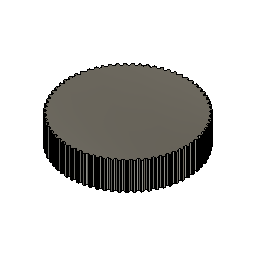
gear_69z (Autodesk Fusion 360 design; units mm, degrees)
Autodesk Fusion 360 part; units mm, degrees
sketch "Sketch1" plane through (0, 0, 0) normal (0, 0, 1) x (1, 0, 0) in component "gt2 pulley"
  circle A0 centre (0, 0) radius 21.9634 construction
  circle A1 centre (0, 0) radius 20.9594 construction
  line L0 (0, 0) -> (0, 21.9634) construction
  line L1 (0, 0) -> (0.9997, 21.9406) construction
  line L2 (0, 0) -> (1.4056, 21.9184) construction
  circle A2 centre (0, 0) radius 21.7094 construction
  arc A3 (0.3936, 21.5719) -> (0.4678, 21.2766) centre (1.3893, 21.6649) ccw
  circle A4 centre (0, 0) radius 21.5594 construction
  arc A5 (0.2459, 21.708) -> (0, 21.7094) centre (0, 0) ccw
  arc A6 (0.3936, 21.5719) -> (0.2459, 21.708) centre (0.2443, 21.558) ccw
  arc A7 (0.4678, 21.2766) -> (0.954, 20.9377) centre (0.9792, 21.4921) ccw
  arc A8 (0, 21.7094) -> (-0.2459, 21.708) centre (0, 0) ccw
  arc A9 (-0.2459, 21.708) -> (-0.3936, 21.5719) centre (-0.2443, 21.558) ccw
  arc A10 (-0.4678, 21.2766) -> (-0.3936, 21.5719) centre (-1.3893, 21.6649) ccw
  arc A11 (-0.954, 20.9377) -> (-0.4678, 21.2766) centre (-0.9792, 21.4921) ccw
  arc A12 (0.954, 20.9377) -> (-0.954, 20.9377) centre (0, 0) ccw
  point P0 (1.3893, 21.6649)
  point P1 (0, 21.7094)
  dimension "d18" = 43.9268
  dimension "d19" = 2.609
  dimension "d22" = 1.004
  dimension "d24" = 0.75
  dimension "d26" = 1
  dimension "d27" = 0.15
  dimension "d28" = 0.15
  dimension "d47" = 0.555
  dimension "d52" = 3.812
  constraint coincident A0.centre A1.centre
  constraint coincident A0 L0.end
  constraint vertical L0
  constraint coincident A0 L1.end
  constraint coincident A0 L2.end
  constraint concentric A1 A2
  constraint coincident A1 A7.end
  constraint coincident L1 A7.end
  constraint coincident A2 P0
  constraint coincident L2 P0
  constraint coincident P0 A3.centre
  constraint coincident A2 P1
  constraint coincident L0 P1
  constraint concentric A2 A4
  constraint coincident P1 A5.end
  constraint coincident A4 A6.centre
  constraint coincident A3.start A6.start
  constraint tangent A3 A6
  constraint tangent A3 A7
  constraint symmetric L0 A7.end A11.start
  constraint symmetric L0 A3.start A9.end
  constraint symmetric L0 A3.end A10.start
  constraint symmetric L0 A3 A10
  constraint symmetric L0 A5.start A8.end
  constraint symmetric L0 P1 A5.end
  constraint symmetric L0 A5 A8
  constraint symmetric L0 A6 A9
  constraint symmetric L0 A7 A11
  constraint coincident A1 A11.start
  constraint tangent A1 A7
  constraint coincident L1 A7.centre
  measures "d18" diameter of A0
  measures "d19" angle of L0 L1
  measures "d22" distance of A0 A1
  measures "d24" distance of A1 A2
  measures "d26" radius of A3
  measures "d27" distance of A2 A4
  measures "d28" radius of A6
  measures "d47" radius of A7
extrude "Extrude1" add sketch "Sketch1" along normal blind 10 makes body 1
pattern_circular "C-Pattern1" count 69 over 360 about axis through (0, 0, 1.75) along (0, 0, 1) of bodies 1 makes body 2 at (-1.1657, 20.9269, 3.3333) makes body 3 at (-3.9003, 20.5933, 6.6667) makes body 4 at (-6.3658, 19.9693, 6.6667) makes body 5 at (-8.1553, 19.3077, 6.6667) makes body 6 at (-9.8773, 18.4861, 6.6667) makes body 7 at (-10.9806, 17.8528, 6.6667) makes body 8 at (-13.062, 16.3914, 6.6667) makes body 9 at (-13.391, 16.1238, 3.3333) makes body 10 at (-15.6748, 13.9139, 6.6667) makes body 11 at (-17, 12.2595, 6.6667) makes body 12 at (-18.0444, 10.6628, 6.6667) makes body 13 at (-18.9393, 8.9778, 6.6667) makes body 14 at (-19.117, 8.5927, 3.3333) makes body 15 at (-20.2521, 5.3991, 6.6667) makes body 16 at (-20.3572, 4.9882, 3.3333) makes body 17 at (-20.7264, 3.1163, 3.3333) makes body 18 at (-20.9239, 1.2187, 6.6667) makes body 19 at (-20.903, -1.5361, 6.6667) makes body 20 at (-20.7104, -3.2212, 6.6667) makes body 21 at (-20.3317, -5.0911, 6.6667) makes body 22 at (-19.9853, -6.3152, 3.3333) makes body 23 at (-19.0733, -8.6893, 6.6667) makes body 24 at (-17.7689, -11.1158, 6.6667) makes body 25 at (-17.5404, -11.473, 3.3333) makes body 26 at (-16.4244, -13.0205, 6.6667) makes body 27 at (-15.1723, -14.4601, 3.3333) makes body 28 at (-13.7946, -15.7799, 3.3333) makes body 29 at (-12.3025, -16.969, 3.3333) makes body 30 at (-9.9707, -18.4359, 6.6667) makes body 31 at (-7.8614, -19.4292, 6.6667) makes body 32 at (-5.8587, -20.1239, 6.6667) makes body 33 at (-5.4503, -20.2383, 3.3333) makes body 34 at (-3.5873, -20.6501, 3.3333) makes body 35 at (-1.6947, -20.8908, 3.3333) makes body 36 at (1.6947, -20.8908, 6.6667) makes body 37 at (3.5873, -20.6501, 6.6667) makes body 38 at (4.8336, -20.3944, 6.6667) makes body 39 at (7.2681, -19.6589, 6.6667) makes body 40 at (8.8338, -19.0068, 6.6667) makes body 41 at (10.1567, -18.3341, 6.6667) makes body 42 at (11.7818, -17.3345, 6.6667) makes body 43 at (13.3093, -16.1913, 6.6667) makes body 44 at (14.111, -15.4976, 3.3333) makes body 45 at (15.4618, -14.1502, 6.6667) makes body 46 at (17.1841, -12.0001, 6.6667) makes body 47 at (17.7689, -11.1158, 3.3333) makes body 48 at (18.7061, -9.4539, 6.6667) makes body 49 at (19.9853, -6.3152, 6.6667) makes body 50 at (20.2791, -5.2966, 6.6667) makes body 51 at (20.6767, -3.4305, 6.6667) makes body 52 at (20.8468, -2.1698, 3.3333) makes body 53 at (20.9577, -0.2651, 3.3333) makes body 54 at (20.895, 1.6418, 3.3333) makes body 55 at (20.3572, 4.9882, 6.6667) makes body 56 at (20.017, 6.2141, 6.6667) makes body 57 at (19.117, 8.5927, 6.6667) makes body 58 at (18.9393, 8.9778, 3.3333) makes body 59 at (18.0444, 10.6628, 3.3333) makes body 60 at (17, 12.2595, 6.6667) makes body 61 at (15.39, 14.2282, 6.6667) makes body 62 at (13.8742, 15.7099, 6.6667) makes body 63 at (11.8693, 17.2747, 6.6667) makes body 64 at (10.2493, 18.2824, 6.6667) makes body 65 at (8.5443, 19.1387, 6.6667) makes body 66 at (7.3674, 19.6218, 6.6667) makes body 67 at (5.5526, 20.2105, 6.6667) makes body 68 at (4.5235, 20.4654, 3.3333) makes body 69 at (1.8003, 20.8819, 6.6667)
sketch "Sketch2" plane through (0, 0, 10) normal (0, 0, 1) x (-1, 0, 0)
  arc A0 (-13.1544, -17.1016) -> (-13.1167, -17.2989) centre (-13.0261, -17.1793) ccw
  arc A1 (-13.1167, -17.2989) -> (-12.7214, -17.5916) centre (0, 0) ccw
  arc A2 (-12.7214, -17.5916) -> (-12.5217, -17.5701) centre (-12.6335, -17.4701) ccw
  arc A3 (-12.2864, -17.3769) -> (-12.5217, -17.5701) centre (-11.7769, -18.2374) ccw
  arc A4 (-11.694, -17.3939) -> (-12.2864, -17.3769) centre (-12.0036, -17.8545) ccw
  arc A5 (-13.2272, -16.2584) -> (-11.694, -17.3939) centre (0, 0) ccw
  arc A6 (-13.0382, -16.8201) -> (-13.2272, -16.2584) centre (-13.5775, -16.6889) ccw
  arc A7 (-13.1544, -17.1016) -> (-13.0382, -16.8201) centre (-14.0099, -16.5838) ccw
  circle A8 centre (0, 0) radius 20.9594
  constraint coincident A1.centre A5.centre
extrude "Extrude2" add sketch "Sketch2" against normal blind 10 contours A5 A8 bodies 1 2 3 4 5 6 7 8 9 10 11 12 13 14 15 16 17 18 19 20 21 22 23 24 25 26 27 28 29 30 31 32 33 34 35 36 37 38 39 40 41 42 43 44 45 46 47 48 49 50 51 52 53 54 55 56 57 58 59 60 61 62 63 64 65 66 67 68 69
extrude "Extrude4" [suppressed] in component "gt2 pulley"
pattern_circular "C-Pattern7" [suppressed] in component "gt2 pulley"
extrude "Extrude3" [suppressed] in component "gt2 pulley"
pattern_circular "C-Pattern6" [suppressed] in component "gt2 pulley"
extrude "Extrude2'" [suppressed] in component "gt2 pulley"
pattern_circular "C-Pattern5" [suppressed] in component "gt2 pulley"
extrude "Extrude1'" [suppressed] in component "gt2 pulley"
pattern_circular "C-Pattern4" [suppressed] in component "gt2 pulley"
pattern_circular "C-Pattern3" [suppressed] in component "gt2 pulley"
pattern_circular "C-Pattern2" [suppressed] in component "gt2 pulley"
pattern_circular "C-Pattern1'" [suppressed] in component "gt2 pulley"
copy_body "Body->Comp1" [suppressed] in component "Component"
copy_body "Body->Comp2" [suppressed] in component "Component'"
copy_body "Body->Comp3" [suppressed] in component "Component''"
copy_body "Body->Comp4" [suppressed] in component "Component'''"
copy_body "Body->Comp5" [suppressed] in component "Component''''"
copy_body "Body->Comp6" [suppressed] in component "Component'''''"
copy_body "Body->Comp7" [suppressed] in component "Component''''''"
copy_body "Body->Comp8" [suppressed] in component "Component'''''''"
copy_body "Body->Comp9" [suppressed] in component "Component''''''''"
copy_body "Body->Comp10" [suppressed] in component "Component'''''''''"
copy_body "Body->Comp11" [suppressed] in component "Component''''''''''"
copy_body "Body->Comp12" [suppressed] in component "Component'''''''''''"
copy_body "Body->Comp13" [suppressed] in component "Component''''''''''''"
copy_body "Body->Comp14" [suppressed] in component "Component'''''''''''''"
copy_body "Body->Comp15" [suppressed] in component "Component''''''''''''''"
copy_body "Body->Comp16" [suppressed] in component "Component'''''''''''''''"
copy_body "Body->Comp17" [suppressed] in component "Component''''''''''''''''"
copy_body "Body->Comp18" [suppressed] in component "Component'''''''''''''''''"
copy_body "Body->Comp19" [suppressed] in component "Component''''''''''''''''''"
copy_body "Body->Comp20" [suppressed] in component "Component'''''''''''''''''''"
component "gt2 pulley" placed x (1, 0, 0) y (0, 1, 0) z (0, 0, 1) at (0, 0, 0)
equation "NumTeeth = 69" comment "min 20"
equation "ToothPitch = 2 mm"
equation "PullyDia = NumTeeth * ToothPitch / PI"
equation "ToothAng = ( ( 360 / NumTeeth ) * 1 deg )"
equation "TransOffsetAngle = ToothAng * 0.2"
equation "Sholulder_Radius = 0.15 mm"
equation "Root_Radius = 0.555 mm"
equation "TransRadius = 1 mm"
equation "ToolHeight = 0.75 mm"
equation "PLD = 0.254 mm"
equation "d18 = PullyDia"
equation "d19 = ToothAng / 2"
equation "d22 = PLD + ToolHeight"
equation "d24 = ToolHeight"
equation "d26 = TransRadius"
equation "d27 = Sholulder_Radius"
equation "d31 = NumTeeth"
equation "d33 = NumTeeth"
equation "d35 = NumTeeth"
equation "d37 = NumTeeth"
equation "d41 = NumTeeth"
equation "d45 = NumTeeth"
equation "d47 = Root_Radius"
equation "d50 = NumTeeth"
